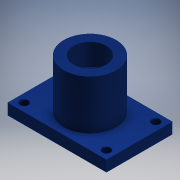
# Autodesk Inventor part: SoporteVarillaZ
Saved by Autodesk Inventor 2018 (Build 220112000, 112)
## iProperties
Created: 2018-03-10
Part Number: SoporteVarillaZ
Material: Genérico
Document SubType Name: Modeling
Designer: Carlos
Density: 1 g/cm^3
Appearance: Anodizado - Azul
Author: Carlos
Autodesk Inventor part; units mm, degrees
ref_plane "YZ Plane" through (0, 0, 0) normal (1, 0, 0) x (0, 1, 0)
ref_plane "XZ Plane" through (0, 0, 0) normal (0, 1, 0) x (-1, 0, 0)
ref_plane "XY Plane" through (0, 0, 0) normal (0, 0, 1) x (1, 0, 0)
sketch "Boceto1" plane through (0, 0, 0) normal (0, 0, 1) x (1, 0, 0)
  line L0 (-18, -12) -> (18, -12)
  line L1 (18, -12) -> (18, 12)
  line L2 (18, 12) -> (-18, 12)
  line L3 (-18, 12) -> (-18, -12)
  line L4 (-18, -12) -> (18, 12) construction
  line L5 (18, -12) -> (-18, 12) construction
  circle A0 centre (0, 0) radius 9.525
  line L6 (-15, -9) -> (15, -9)
  line L7 (15, -9) -> (15, 9)
  line L8 (15, 9) -> (-15, 9)
  line L9 (-15, 9) -> (-15, -9)
  line L10 (-15, -9) -> (15, 9) construction
  line L11 (15, -9) -> (-15, 9) construction
  dimension "d0" = 36
  dimension "d1" = 24
  dimension "d2" = 19.05
  dimension "d3" = 30
  dimension "d4" = 18
  constraints: 24 end point, 4 midpoint, 4 parallel, 2 horizontal, 2 perpendicular, 1 centre point, 1 coincident
  measures "d0" distance of L1.end L2.end
  measures "d1" distance of L0.end L1.end
  measures "d2" diameter of A0
  measures "d3" distance of L8.end L7.end
  measures "d4" distance of L6.end L7.end
extrude "Extrusión1" add sketch "Boceto1" along normal blind 4 contours L3 L2 L1 L0 | A0 L6 L8 | A0 L8 L7 L6 | L8 A0 | A0 L6 | A0 L6 L9 L8
sketch "Boceto2" plane through (0, 0, 4) normal (0, 0, 1) x (1, 0, 0)
  circle A0 centre (0, 0) radius 9.525
  dimension "d7" = 19.05
  constraints: 1 centre point, 1 coincident
  measures "d7" diameter of A0
extrude "Extrusión2" add sketch "Boceto2" along normal blind 18
sketch "Boceto3" plane through (0, 0, 22) normal (0, 0, 1) x (1, 0, 0)
  point P0 (0, 0)
  point P1 (0, 0)
  constraints: 1 coincident
hole "Agujero1" at (0, 0, 22) direction (0, 0, -1) diameter 12 depth 8
sketch "Boceto4" plane through (0, 0, 0) normal (0, 0, -1) x (-1, 0, 0)
  line L0 (15, -9) -> (-15, -9)
  line L1 (-15, -9) -> (-15, 9)
  line L2 (-15, 9) -> (15, 9)
  line L3 (15, 9) -> (15, -9)
  line L4 (15, -9) -> (-15, 9) construction
  line L5 (-15, -9) -> (15, 9) construction
  point P0 (0, 0)
  dimension "d17" = 30
  dimension "d18" = 18
  constraints: 12 end point, 2 midpoint, 2 parallel, 1 horizontal, 1 perpendicular
  measures "d17" distance of L1.end L2.end
  measures "d18" distance of L0.end L1.end
hole "Agujero2" at (15, 9, 0) at (15, -9, 0) at (-15, 9, 0) at (-15, -9, 0) direction (0, 0, 1) diameter 3 depth 8 tip angle 118
